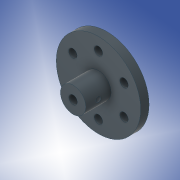
# Autodesk Inventor part: BA008
Saved by Autodesk Inventor 2017 (Build 210142000, 142)
## iProperties
Created: 2017-06-15
Part Number: BA008
Material: ABS Plastic
Document SubType Name: Modeling
Designer: zallen
Density: 1.06 g/cm^3
Appearance: CR Dark Blue
Author: zallen
Autodesk Inventor part; units mm, degrees
ref_plane "YZ Plane" through (0, 0, 0) normal (1, 0, 0) x (0, 1, 0)
ref_plane "XZ Plane" through (0, 0, 0) normal (0, 1, 0) x (-1, 0, 0)
ref_plane "XY Plane" through (0, 0, 0) normal (0, 0, 1) x (1, 0, 0)
sketch "Sketch1" plane through (0, 0, 0) normal (0, 0, 1) x (1, 0, 0)
  circle A0 centre (0, 0) radius 25
  circle A1 centre (0, 17.5) radius 2.5
  circle A2 centre (0, 0) radius 17.5 construction
  circle A3 centre (-15.1554, 8.75) radius 2.5
  circle A4 centre (-15.1554, -8.75) radius 2.5
  circle A5 centre (0, -17.5) radius 2.5
  circle A6 centre (15.1554, -8.75) radius 2.5
  circle A7 centre (15.1554, 8.75) radius 2.5
  circle A8 centre (0, 0) radius 2.5
  dimension "d2" = 35
  dimension "d0" = 50
  dimension "d1" = 5
  dimension "d5" = 360
  dimension "d7" = 5
  constraints: 8 centre point, 3 coincident, 2 vertical alignment, 15 other
  measures "d0" diameter of A0
  measures "d1" diameter of A1
  measures "d7" diameter of A8
extrude "Extrusion1" add sketch "Sketch1" along normal blind 5
sketch "Sketch2" plane through (0, 0, 5) normal (0, 0, 1) x (1, 0, 0)
  circle A0 centre (0, 0) radius 2.5 projected
  circle A1 centre (0, 0) radius 7.5
  dimension "d10" = 5
  constraints: 1 centre point
  measures "d10" radial gap between concentric circles of A0 A1
extrude "Extrusion2" add sketch "Sketch2" along normal blind 15
sketch "Sketch3" plane through (0, 0, 0) normal (1, 0, 0) x (0, 1, 0)
  circle A0 centre (0, 12.5) radius 1.5
  point P0 (0, 0)
  dimension "d13" = 3
  dimension "d14" = 12.5
  constraints: 1 centre point, 1 vertical alignment
  measures "d13" diameter of A0
  measures "d14" distance of point (0, 0) A0.centre
extrude "Extrusion3" cut sketch "Sketch3" along normal blind 10
body "Solid1"
